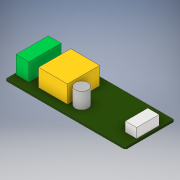
# Autodesk Inventor part: PZEM-00ET
Saved by Autodesk Inventor 2019 (Build 230136000, 136)
## iProperties
Created: 2022-02-03
Part Number: PZEM-00ET
Material: Generic
Document SubType Name: Modeling
Designer: josec
Density: 1 g/cm^3
Appearance: Default
Author: josec
Autodesk Inventor part; units mm, degrees
ref_plane "YZ Plane" through (0, 0, 0) normal (1, 0, 0) x (0, 1, 0)
ref_plane "XZ Plane" through (0, 0, 0) normal (0, 1, 0) x (-1, 0, 0)
ref_plane "XY Plane" through (0, 0, 0) normal (0, 0, 1) x (1, 0, 0)
sketch "Sketch1" plane through (0, 0, 0) normal (0, 1, 0) x (-1, 0, 0)
  line L0 (0, 0) -> (-74, 0)
  line L1 (-74, 0) -> (-74, -30)
  line L2 (-74, -30) -> (0, -30)
  line L3 (0, -30) -> (0, 0)
  dimension "d0" = 74
  dimension "d1" = 30
  constraints: 8 end point, 2 parallel, 1 horizontal, 1 perpendicular
  measures "d0" distance of L2.end L1.end
  measures "d1" distance of L1.end L0.end
extrude "Extrusion1" add sketch "Sketch1" along normal blind 1.5
sketch "Sketch2" plane through (0, 1.5, 0) normal (0, 1, 0) x (1, 0, 0)
  line L0 (0, 0) -> (74, 0) construction
  line L1 (0, 0) -> (0, 5) construction
  line L2 (0, 30) -> (0, 0) construction
  line L3 (0, 30) -> (0, 25) construction
  line L4 (0, 25) -> (42, 25)
  line L5 (42, 25) -> (42, 5)
  line L6 (42, 5) -> (0, 5)
  line L7 (0, 5) -> (0, 25)
  dimension "d4" = 5
  dimension "d5" = 5
  dimension "d6" = 42
  constraints: 12 end point, 2 parallel, 2 point on line, 1 horizontal, 1 perpendicular
  measures "d4" distance of L0.start L1.end
  measures "d5" distance of L2.start L3.end
  measures "d6" distance of L5.end L6.end
extrude "Extrusion2" add sketch "Sketch2" along normal blind 11
sketch "Sketch3" plane through (0, 1.5, 0) normal (0, 1, 0) x (1, 0, 0)
  line L0 (74, 30) -> (0, 30) construction
  line L1 (74, 30) -> (74, 22) construction
  line L2 (74, 0) -> (74, 30) construction
  line L3 (0, 0) -> (74, 0) construction
  line L4 (74, 0) -> (74, 8) construction
  line L5 (74, 22) -> (66, 22)
  line L6 (66, 22) -> (66, 8)
  line L7 (66, 8) -> (74, 8)
  line L8 (74, 8) -> (74, 22)
  dimension "d9" = 8
  dimension "d10" = 8
  dimension "d11" = 8
  constraints: 12 end point, 2 parallel, 2 point on line, 1 horizontal, 1 perpendicular
  measures "d9" distance of L0.start L1.end
  measures "d10" distance of L2.start L4.end
  measures "d11" distance of L7.end L6.end
extrude "Extrusion3" add sketch "Sketch3" along normal blind 6
sketch "Sketch4" plane through (0, 12.5, 0) normal (0, 1, 0) x (1, 0, 0)
  line L0 (0, 25) -> (42, 25) projected
  line L1 (42, 5) -> (0, 5) projected
  line L2 (0, 25) -> (9, 25)
  line L3 (9, 25) -> (9, 5)
  line L4 (9, 5) -> (0, 5)
  line L5 (0, 5) -> (0, 25)
  line L6 (0, 25) -> (32, 25)
  line L7 (32, 25) -> (32, 5)
  line L8 (32, 5) -> (0, 5)
  line L9 (0, 5) -> (0, 25)
  line L10 (32, 25) -> (15, 25)
  line L11 (15, 25) -> (15, 5)
  line L12 (15, 5) -> (32, 5)
  line L13 (32, 5) -> (32, 25)
  point P0 (0, 0)
  dimension "d14" = 9
  dimension "d15" = 32
  dimension "d16" = 17
  constraints: 24 end point, 6 parallel, 3 horizontal, 3 perpendicular, 3 point on line
  measures "d14" distance of L3.end L4.end
  measures "d15" distance of L7.end L8.end
  measures "d16" distance of L12.end L11.end
extrude "Extrusion4" cut sketch "Sketch4" against normal up to surface (11 mm away) contours L0 L11 L1 L3
sketch "Sketch5" plane through (0, 12.5, 0) normal (0, 1, 0) x (1, 0, 0)
  line L0 (15, 5) -> (42, 5) projected
  line L1 (15, 25) -> (33, 25)
  line L2 (33, 25) -> (33, 5)
  line L3 (33, 5) -> (15, 5)
  line L4 (15, 5) -> (15, 25)
  line L5 (42, 25) -> (33, 25)
  line L6 (33, 25) -> (33, 5)
  line L7 (33, 5) -> (42, 5)
  line L8 (42, 5) -> (42, 25)
  point P0 (0, 0)
  dimension "d19" = 18
  constraints: 16 end point, 4 parallel, 2 horizontal, 2 perpendicular, 1 point on line
  measures "d19" distance of L2.end L3.end
extrude "Extrusion5" cut sketch "Sketch5" against normal up to surface (11 mm away) contours L2 L5 L8 L0
sketch "Sketch6" plane through (0, 1.5, 0) normal (0, 1, 0) x (1, 0, 0)
  line L0 (0, 25) -> (9, 25) construction
  line L1 (0, 25) -> (42, 25) construction
  line L2 (42, 25) -> (42, 5) construction
  line L3 (42, 5) -> (0, 5) construction
  line L4 (0, 5) -> (0, 25) construction
  circle A0 centre (37.6164, 9.2055) radius 4
  point P0 (0, 0)
  dimension "d22" = 42
  dimension "d23" = 20
  dimension "d24" = 8
  constraints: 8 end point, 2 parallel, 1 centre point, 1 horizontal, 1 perpendicular
  measures "d22" distance of L2.end L3.end
  measures "d23" distance of L1.end L2.end
  measures "d24" diameter of A0
extrude "Extrusion6" add sketch "Sketch6" along normal blind 10
sketch "Sketch7" plane through (74, 0, 0) normal (1, 0, 0) x (0, 0, -1)
  point P0 (0, 0)
sketch "Sketch8" plane through (0, 0, -30) normal (-1, 0, 0) x (0, 0, 1)
  line L0 (25, 1.5) -> (25, 12.5) projected
  line L1 (25, 1.5) -> (5, 1.5) projected
  line L2 (25, 12.5) -> (5, 12.5)
  line L3 (5, 12.5) -> (5, 1.5)
  line L4 (5, 1.5) -> (25, 1.5)
  line L5 (25, 1.5) -> (25, 12.5)
  point P0 (30, 0)
  constraints: 8 end point, 2 parallel, 1 horizontal, 1 perpendicular
extrude "Extrusion7" cut sketch "Sketch8" against normal blind 1
sketch "Sketch9" plane through (74, 0, 0) normal (1, 0, 0) x (0, 0, -1)
  line L0 (8, 1.5) -> (8, 7.5) projected
  line L1 (22, 1.5) -> (22, 7.5) projected
  line L2 (8, 7.5) -> (22, 7.5)
  line L3 (22, 7.5) -> (22, 1.5)
  line L4 (22, 1.5) -> (8, 1.5)
  line L5 (8, 1.5) -> (8, 7.5)
  point P0 (0, 0)
  constraints: 8 end point, 2 parallel, 1 horizontal, 1 perpendicular
extrude "Extrusion8" cut sketch "Sketch9" against normal blind 1
body "Solid1"
